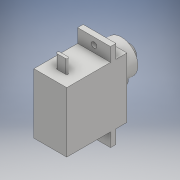
# Autodesk Inventor part: towerpro
Saved by Autodesk Inventor 2017 (Build 210142000, 142)
## iProperties
Created: 2017-05-10
Part Number: towerpro
Material: Ogólny
Document SubType Name: Modeling
Designer: Damian
Density: 1 g/cm^3
Appearance: Domyślna
Author: Damian
Autodesk Inventor part; units mm, degrees
ref_plane "YZ Plane" through (0, 0, 0) normal (1, 0, 0) x (0, 1, 0)
ref_plane "XZ Plane" through (0, 0, 0) normal (0, 1, 0) x (-1, 0, 0)
ref_plane "XY Plane" through (0, 0, 0) normal (0, 0, 1) x (1, 0, 0)
sketch "Szkic1" plane through (0, 0, 0) normal (0, 1, 0) x (-1, 0, 0)
  line L0 (0, 0) -> (12, 0)
  line L1 (12, 0) -> (12, 22)
  line L2 (12, 22) -> (0, 22)
  line L3 (0, 22) -> (0, 0)
  dimension "d0" = 12
  dimension "d1" = 22
  constraints: 8 end point, 2 parallel, 1 horizontal, 1 perpendicular
  measures "d0" distance of L2.end L1.end
  measures "d1" distance of L1.end L0.end
extrude "Wyciągnięcie proste1" add sketch "Szkic1" along normal blind 22
sketch "Szkic2" plane through (-12, 0, 22) normal (0, 0, 1) x (1, 0, 0)
  line L0 (0, 0) -> (0, 22) projected
  line L1 (12, 0) -> (12, 22) projected
  line L2 (0, 18) -> (12, 18)
  line L3 (12, 18) -> (12, 16)
  line L4 (12, 16) -> (0, 16)
  line L5 (0, 16) -> (0, 18)
  line L6 (0, 22) -> (12, 22) projected
  dimension "d4" = 2
  dimension "d5" = 4
  constraints: 8 end point, 2 parallel, 2 point on line, 1 horizontal, 1 perpendicular
  measures "d4" distance between parallel lines of L4 L2
  measures "d5" distance between parallel lines of L2 L6
extrude "Wyciągnięcie proste2" add sketch "Szkic2" along normal blind 5 contours L0 L2 L1 L4
sketch "Szkic3" plane through (0, 0, 0) normal (0, 0, -1) x (-1, 0, 0)
  line L0 (0, 16) -> (0, 18) projected
  line L1 (12, 16) -> (0, 16) projected
  line L2 (0, 18) -> (12, 18)
  line L3 (12, 18) -> (12, 16)
  line L4 (12, 16) -> (0, 16)
  line L5 (0, 16) -> (0, 18)
  point P0 (0, 0)
  constraints: 8 end point, 2 parallel, 1 horizontal, 1 perpendicular
extrude "Wyciągnięcie proste3" add sketch "Szkic3" along normal blind 5
sketch "Szkic4" plane through (-12, 18, 0) normal (0, 1, 0) x (1, 0, 0)
  line L0 (0, 5) -> (12, 5) projected
  point P0 (12, 0)
  point P1 (6, 2.5)
  point P2 (6, -24.839)
  dimension "d10" = 2.5
  measures "d10" distance from line of L0 point (6, 2.5)
hole "Otwór1" at (-6, 18, -2.5) direction (0, -1, 0) diameter 2 end through all
sketch "Szkic5" plane through (-12, 18, 22) normal (0, 1, 0) x (1, 0, 0)
  line L0 (12, -5) -> (0, -5) projected
  point P0 (12, 22)
  point P1 (6, -2.5)
  dimension "d18" = 2.5
  measures "d18" distance from line of L0 point (6, -2.5)
hole "Otwór2" at (-6, 18, 24.5) direction (0, -1, 0) diameter 2 end through all
sketch "Szkic6" plane through (0, 22, 0) normal (0, 1, 0) x (1, 0, 0)
  line L0 (-12, -22) -> (0, -22) projected
  arc A0 (-8.3077, -10.4615) -> (-3.6923, -10.4615) centre (-6, -16) ccw
  line L1 (0, 0) -> (-12, 0) projected
  arc A1 (-3.6923, -10.4615) -> (-8.3077, -10.4615) centre (-6, -9.5) ccw
  dimension "d26" = 6
  dimension "d27" = 9.5
  dimension "d28" = 5
  constraints: 4 point on circle, 2 centre point, 2 coincident
  measures "d26" distance from line of L0 point (-6, -16)
  measures "d27" distance from line of L1 point (-6, -9.5)
  measures "d28" diameter of A1
extrude "Wyciągnięcie proste4" add sketch "Szkic6" along normal blind 4
sketch "Szkic7" plane through (0, 26, 0) normal (0, 1, 0) x (1, 0, 0)
  circle A0 centre (-6, -16) radius 2.5
  arc A1 (-8.3077, -10.4615) -> (-3.6923, -10.4615) centre (-6, -16) ccw projected
  point P0 (0, 0)
  dimension "d31" = 5
  constraints: 1 centre point, 1 concentric
  measures "d31" diameter of A0
extrude "Wyciągnięcie proste5" add sketch "Szkic7" along normal blind 3
sketch "Szkic8" plane through (-12, 0, 22) normal (0, 0, 1) x (1, 0, 0)
  line L0 (4.5, 4) -> (7.5, 4)
  line L1 (8, 4.5) -> (8, 4.5)
  line L2 (7.5, 5) -> (4.5, 5)
  line L3 (4, 4.5) -> (4, 4.5)
  line L4 (0, 0) -> (12, 0) projected
  line L5 (12, 0) -> (12, 16) projected
  arc A0 (4.5, 5) -> (4, 4.5) centre (4.5, 4.5) ccw
  arc A1 (4, 4.5) -> (4.5, 4) centre (4.5, 4.5) ccw
  arc A2 (8, 4.5) -> (7.5, 5) centre (7.5, 4.5) ccw
  arc A3 (7.5, 4) -> (8, 4.5) centre (7.5, 4.5) ccw
  point P0 (8, 5)
  point P1 (8, 4)
  point P2 (4, 5)
  dimension "d34" = 4
  dimension "d35" = 1
  dimension "d36" = 4
  dimension "d37" = 4
  dimension "d38" = 0.5
  constraints: 8 end point, 8 point on circle, 8 tangent, 6 point on line, 4 centre point, 3 equal radius, 2 parallel, 1 horizontal, 1 perpendicular
  measures "d34" distance of point (4, 5) point (8, 5)
  measures "d35" distance of point (8, 5) point (8, 4)
  measures "d36" distance between parallel lines of L4 L0
  measures "d37" distance between parallel lines of L5 L1
  measures "d38" radius of A0
extrude "Wyciągnięcie proste6" add sketch "Szkic8" along normal blind 5
